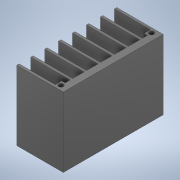
# Autodesk Inventor part: HS117-30
Saved by Autodesk Inventor 2020 (Build 240168000, 168)
## iProperties
Created: 2021-05-17
Part Number: HS117-30
Material: Типовые
Document SubType Name: Modeling
Designer: Михаил
Density: 1 g/cm^3
Appearance: По умолчанию
Author: Михаил
Autodesk Inventor part; units mm, degrees
ref_plane "YZ Plane" through (0, 0, 0) normal (1, 0, 0) x (0, 1, 0)
ref_plane "XZ Plane" through (0, 0, 0) normal (0, 1, 0) x (-1, 0, 0)
ref_plane "XY Plane" through (0, 0, 0) normal (0, 0, 1) x (1, 0, 0)
sketch "Эскиз1" plane through (0, 0, 0) normal (0, 1, 0) x (-1, 0, 0)
  line L0 (17, 0) -> (17, -1)
  line L1 (0, -6) -> (17, -6)
  line L2 (17, -6) -> (17, -7)
  line L3 (17, -7) -> (0, -7)
  line L4 (0, -12) -> (17, -12)
  line L5 (17, -12) -> (17, -13)
  line L6 (17, -13) -> (0, -13)
  line L7 (0, -18) -> (17, -18)
  line L8 (17, -18) -> (17, -19)
  line L9 (17, -19) -> (0, -19)
  line L10 (0, -24) -> (17, -24)
  line L11 (17, -24) -> (17, -25)
  line L12 (17, -25) -> (0, -25)
  line L13 (0, -30) -> (17, -30)
  line L14 (17, -30) -> (17, -31)
  line L15 (17, -31) -> (0, -31)
  line L16 (0, -36) -> (17, -36)
  line L17 (17, -36) -> (17, -37)
  line L18 (17, -37) -> (0, -37)
  line L19 (17, -43) -> (17, -42)
  line L20 (0, -7) -> (0, -12)
  line L21 (0, -13) -> (0, -18)
  line L22 (0, -19) -> (0, -24)
  line L23 (0, -25) -> (0, -30)
  line L24 (0, -31) -> (0, -36)
  line L25 (1.5, -1) -> (1.5, -3.8)
  line L26 (1.5, -3.8) -> (0, -3.8)
  line L27 (0, -3.8) -> (0, -6)
  line L28 (1.5, -1) -> (17, -1)
  line L29 (-3, 0) -> (-3, -43)
  line L30 (0, -37) -> (0, -39.2)
  line L31 (0, -39.2) -> (1.5, -39.2)
  line L32 (1.5, -39.2) -> (1.5, -42)
  line L33 (1.5, -42) -> (17, -42)
  line L34 (-3, 0) -> (17, 0)
  line L35 (17, -43) -> (-3, -43)
  point P0 (0, 0)
  dimension "d46" = 43
  dimension "d47" = 3
  dimension "d48" = 3
  dimension "d49" = 20
  dimension "d50" = 4.5
  dimension "d51" = 4.5
  dimension "d52" = 3.8
  dimension "d53" = 20
  dimension "d54" = 1
  dimension "d55" = 3.8
  dimension "d56" = 3
  dimension "d57" = 3
  dimension "d58" = 3
  dimension "d59" = 3
  dimension "d60" = 3
  dimension "d61" = 3
  dimension "d62" = 1
  dimension "d63" = 5
  dimension "d64" = 43
  dimension "d65" = 5
  dimension "d66" = 5
  dimension "d67" = 5
  dimension "d68" = 5
  dimension "d69" = 5
  dimension "d70" = 5
  dimension "d71" = 1
  dimension "d72" = 1
  dimension "d73" = 1
  dimension "d74" = 1
  dimension "d75" = 1
  dimension "d76" = 17
  constraints: 72 end point, 11 equal length, 9 horizontal, 9 perpendicular, 6 point on line, 3 vertical
  measures "d46" distance of L29.start L29.end
  measures "d47" distance between parallel lines of L29 L30
  measures "d48" distance from line of L29 point (0, 0)
  measures "d49" distance of L29.start L0.start
  measures "d50" distance between parallel lines of L25 L29
  measures "d51" distance between parallel lines of L29 L32
  measures "d52" distance between parallel lines of L35 L31
  measures "d53" distance between parallel lines of L19 L29
  measures "d54" distance between parallel lines of L33 L35
  measures "d55" distance between parallel lines of L34 L26
  measures "d56" distance between parallel lines of L29 L27
  measures "d57" distance between parallel lines of L29 L20
  measures "d58" distance between parallel lines of L29 L21
  measures "d59" distance between parallel lines of L29 L22
  measures "d60" distance between parallel lines of L29 L23
  measures "d61" distance between parallel lines of L29 L24
  measures "d62" distance between parallel lines of L18 L16
  measures "d63" distance between parallel lines of L18 L33
  measures "d64" distance from line of point (0, 0) L35
  measures "d65" distance between parallel lines of L1 L28
  measures "d66" distance between parallel lines of L4 L3
  measures "d67" distance between parallel lines of L7 L6
  measures "d68" distance between parallel lines of L10 L9
  measures "d69" distance between parallel lines of L13 L12
  measures "d70" distance between parallel lines of L16 L15
  measures "d71" distance between parallel lines of L15 L13
  measures "d72" distance between parallel lines of L12 L10
  measures "d73" distance between parallel lines of L9 L7
  measures "d74" distance between parallel lines of L6 L4
  measures "d75" distance between parallel lines of L1 L3
  measures "d76" distance from line of point (0, 0) L0
extrude "Выдавливание1" add sketch "Эскиз1" along normal blind 30
sketch "Эскиз3" plane through (0, 30, 0) normal (0, 1, 0) x (1, 0, 0)
  circle A0 centre (0, 2) radius 1
  line L0 (-17, 0) -> (3, 0) projected
  line L1 (3, 0) -> (3, 43) projected
  circle A1 centre (0, 41) radius 1
  line L2 (3, 43) -> (-17, 43) projected
  point P0 (0, 0)
  dimension "d80" = 2
  dimension "d81" = 2
  dimension "d82" = 3
  dimension "d83" = 2
  dimension "d84" = 3
  dimension "d85" = 2
  constraints: 2 centre point
  measures "d80" diameter of A0
  measures "d81" distance from line of L0 A0.centre
  measures "d82" distance from line of L1 A0.centre
  measures "d83" diameter of A1
  measures "d84" distance from line of L1 A1.centre
  measures "d85" distance from line of L2 A1.centre
extrude "Выдавливание2" cut sketch "Эскиз3" against normal blind 30
